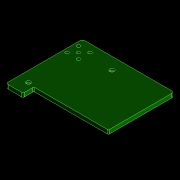
# Autodesk Inventor part: hw_DAA - PCB MicroSD
Saved by Autodesk Inventor 2018 (Build 220112000, 112)
## iProperties
Created: 2024-03-13
Part Number: hw_DAA - PCB MicroSD
Material: PCB
Document SubType Name: Modeling
Designer: cda1
Density: 4 g/cm^3
Appearance: PCB
Author: cda1
Autodesk Inventor part; units mm, degrees
ref_plane "YZ Plane" through (0, 0, 0) normal (1, 0, 0) x (0, 1, 0)
ref_plane "XZ Plane" through (0, 0, 0) normal (0, 1, 0) x (-1, 0, 0)
ref_plane "XY Plane" through (0, 0, 0) normal (0, 0, 1) x (1, 0, 0)
sketch "Boceto1" plane through (0, 0, 0) normal (0, 0, 1) x (1, 0, 0)
  line L0 (-26, 17) -> (26, 17)
  line L1 (26, 17) -> (26, -17)
  line L2 (26, -17) -> (-26, -17)
  line L3 (-26, -17) -> (-26, 17)
  line L4 (-26, 17) -> (26, -17) construction
  line L5 (26, 17) -> (-26, -17) construction
  point P0 (0, 0)
  dimension "d0" = 52
  dimension "d1" = 34
  constraints: 12 end point, 2 midpoint, 2 parallel, 1 horizontal, 1 perpendicular
  measures "d0" distance of L1.end L2.end
  measures "d1" distance of L0.end L1.end
extrude "Extrusión1" add sketch "Boceto1" against normal blind 1.742
fillet "Empalme1" radius 0.5 4 edges at (26, 17, -0.871) (-26, 17, -0.871) (-26, -17, -0.871) (26, -17, -0.871)
sketch "Boceto2" plane through (0, 0, 0) normal (0, 0, 1) x (1, 0, 0)
  line L0 (25.5, 17) -> (-25.5, 17) projected
  line L1 (26, 16.5) -> (26, -16.5) projected
  line L2 (25.5, -17) -> (-25.5, -17) construction
  line L3 (23, -17) -> (-20, -17)
  line L4 (-20, -17) -> (-20, -12.2)
  line L5 (-20, -12.2) -> (23, -12.2)
  line L6 (23, -12.2) -> (23, -17)
  point P0 (0, 0)
  dimension "d13" = 3
  dimension "d14" = 4.8
  dimension "d15" = 43
  constraints: 8 end point, 2 parallel, 1 horizontal, 1 perpendicular, 1 point on line
  measures "d13" distance between parallel lines of L1 L6
  measures "d14" distance of L5.end L3.start
  measures "d15" distance of L4.end L5.end
extrude "Extrusión2" cut sketch "Boceto2" against normal through all
sketch "Boceto3" plane through (0, 0, -1.742) normal (0, 0, -1) x (-1, 0, 0)
  arc A0 (26, 16.5) -> (25.5, 17) centre (25.5, 16.5) ccw projected
  line L0 (26, -16.5) -> (26, 16.5) projected
  arc A1 (25.5, -17) -> (26, -16.5) centre (25.5, -16.5) ccw projected
  line L1 (25.5, 17) -> (27.6, 17)
  line L2 (27.6, 17) -> (27.6, -17)
  line L3 (27.6, -17) -> (25.5, -17)
  point P0 (0, 0)
  dimension "d10" = 1.6
  constraints: 6 end point, 2 perpendicular, 1 horizontal, 1 tangent
  measures "d10" distance between parallel lines of L2 L0
extrude "Extrusión3" add sketch "Boceto3" against normal up to surface (1.742 mm away)
sketch "Boceto4" plane through (0, 0, 0) normal (0, 0, 1) x (1, 0, 0)
  line L0 (-27.6, 17) -> (25.5, 17) construction
  arc A0 (26, 16.5) -> (25.5, 17) centre (25.5, 16.5) ccw construction
  line L1 (26, 16.5) -> (26, -16.5) construction
  line L2 (25.5, -17) -> (23, -17) construction
  arc A1 (25.5, -17) -> (26, -16.5) centre (25.5, -16.5) ccw construction
  line L3 (23, -12.2) -> (23, -17) construction
  line L4 (-20, -12.2) -> (23, -12.2) construction
  line L5 (26, 17) -> (22.8, 17)
  line L6 (22.8, 17) -> (22.8, -17)
  line L7 (22.8, -17) -> (26, -17)
  line L8 (26, -17) -> (26, 17)
  point P0 (0, 0)
  dimension "d16" = 3.2
  dimension "d17" = 34
  constraints: 8 end point, 2 parallel, 2 point on line, 1 horizontal, 1 perpendicular
  measures "d16" distance of L5.start L5.end
  measures "d17" distance of L7.end L5.start
extrude "Extrusión4" cut sketch "Boceto4" against normal up to surface (1.742 mm away)
sketch "Boceto5" plane through (0, 0, 0) normal (0, 0, 1) x (1, 0, 0)
  line L0 (-27.6, 17) -> (22.8, 17) projected
  line L1 (22.8, 17) -> (13.2, 17)
  line L2 (13.2, 17) -> (13.2, -12.2)
  line L3 (13.2, -12.2) -> (22.8, -12.2)
  line L4 (22.8, -12.2) -> (22.8, 17)
  point P0 (0, 0)
  point P1 (22.8, -12.2)
  dimension "d20" = 9.6
  constraints: 8 end point, 2 parallel, 1 coincident, 1 horizontal, 1 perpendicular
  measures "d20" distance between parallel lines of L4 L2
extrude "Extrusión5" cut sketch "Boceto5" against normal up to surface (1.742 mm away)
fillet "Empalme2" radius 1 3 edges at (-27.6, -17, -0.871) (-27.6, 17, -0.871) (13.2, 17, -0.871)
sketch "Boceto8" plane through (0, 0, -1.742) normal (0, 0, -1) x (-1, 0, 0)
  line L0 (20, -17) -> (26.6, -17) projected
  line L1 (20, -12.2) -> (20, -17) projected
  point P0 (0, 0)
  point P1 (22.95, -11.638)
  dimension "d54" = 5.362
  dimension "d55" = 2.95
  measures "d54" distance from line of L0 point (22.95, -11.638)
  measures "d55" distance from line of L1 point (22.95, -11.638)
hole "Agujero3" at (-22.95, -11.638, -1.742) direction (0, 0, 1) diameter 2 end through all countersink diameter 4 countersink angle 90
sketch "Boceto9" plane through (0, 0, -1.742) normal (0, 0, -1) x (-1, 0, 0)
  line L0 (-13.2, 16) -> (-13.2, -12.2) projected
  line L1 (26.6, 17) -> (-12.2, 17) projected
  point P0 (0, 0)
  point P1 (9.05, 11.638)
  dimension "d52" = 22.25
  dimension "d53" = 5.362
  measures "d52" distance from line of L0 point (9.05, 11.638)
  measures "d53" distance from line of L1 point (9.05, 11.638)
hole "Agujero4" at (-9.05, 11.638, -1.742) direction (0, 0, 1) diameter 2 end through all countersink diameter 4 countersink angle 90
sketch "Boceto10" plane through (0, 0, -1.742) normal (0, 0, -1) x (-1, 0, 0)
  line L0 (20.7601, 13.5399) -> (25.8399, 13.5399) construction
  line L1 (25.8399, 13.5399) -> (25.8399, 8.4601) construction
  line L2 (25.8399, 8.4601) -> (20.7601, 8.4601) construction
  line L3 (20.7601, 8.4601) -> (20.7601, 13.5399) construction
  line L4 (20.7601, 13.5399) -> (25.8399, 8.4601) construction
  line L5 (26.6, 17) -> (-12.2, 17) construction
  line L6 (27.6, -16) -> (27.6, 16) construction
  circle A0 centre (20.7601, 13.5399) radius 0.75
  circle A1 centre (25.8399, 13.5399) radius 0.75
  circle A2 centre (20.7601, 8.4601) radius 0.75
  circle A3 centre (25.8399, 8.4601) radius 0.75
  circle A4 centre (23.3, 11) radius 0.7
  point P0 (0, 0)
  dimension "d56" = 7.184
  dimension "d57" = 45
  dimension "d58" = 6
  dimension "d59" = 4.3
  dimension "d60" = 1.5
  dimension "d61" = 1.5
  dimension "d62" = 1.5
  dimension "d63" = 1.5
  dimension "d64" = 1.4
  constraints: 10 end point, 5 centre point, 5 coincident, 2 parallel, 1 horizontal, 1 midpoint, 1 perpendicular
  measures "d56" distance of L0.start L1.end
  measures "d57" angle of L0 L4
  measures "d58" distance from line of L5 point (23.3, 11)
  measures "d59" distance from line of L6 point (23.3, 11)
  measures "d60" diameter of A0
  measures "d61" diameter of A1
  measures "d62" diameter of A2
  measures "d63" diameter of A3
  measures "d64" diameter of A4
extrude "Extrusión6" cut sketch "Boceto10" against normal up to surface (1.742 mm away)
fillet "Empalme3" radius 0.5 1 edges at (13.2, -12.2, -0.871)
fillet "Empalme4" radius 0.5 2 edges at (-20, -17, -0.871) (-20, -12.2, -0.871)
sketch "Boceto11" plane through (0, 0, -1.742) normal (0, 0, -1) x (-1, 0, 0)
  line L0 (-13.2, 17) -> (27.6, 17)
  line L1 (27.6, 17) -> (27.6, 15.258)
  line L2 (27.6, 15.258) -> (-13.2, 15.258)
  line L3 (-13.2, 15.258) -> (-13.2, 17)
  line L4 (-13.2, 16) -> (-13.2, -11.7) projected
  line L5 (27.6, -16) -> (27.6, 16) projected
  line L6 (20, -15.258) -> (27.6, -15.258)
  line L7 (27.6, -15.258) -> (27.6, -17)
  line L8 (27.6, -17) -> (20, -17)
  line L9 (20, -17) -> (20, -15.258)
  line L10 (20, -12.7) -> (20, -16.5) projected
  line L11 (20.5, -17) -> (26.6, -17) projected
  point P0 (0, 0)
  point P1 (26.6, 17)
  dimension "d69" = 1.742
  dimension "d70" = 1.742
  constraints: 16 end point, 6 point on line, 4 parallel, 2 horizontal, 2 perpendicular
  measures "d69" distance of L0.end L1.end
  measures "d70" distance of L6.end L7.end
extrude "Extrusión7" cut sketch "Boceto11" against normal up to surface (1.742 mm away)
fillet "Empalme5" radius 0.5 4 edges at (13.2, 15.258, -0.871) (-27.6, 15.258, -0.871) (-20, -15.258, -0.871) (-27.6, -15.258, -0.871)
